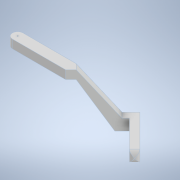
# Autodesk Inventor part: connector
Saved by Autodesk Inventor 2022 (Build 260153000, 153)
## iProperties
Created: 2023-07-22
Part Number: connector
Material: Generic
Document SubType Name: Modeling
Designer: Eric Cao
Density: 1 g/cm^3
Appearance: Plate - Blue
Author: Eric Cao
Autodesk Inventor part; units mm, degrees
ref_plane "YZ Plane" through (0, 0, 0) normal (1, 0, 0) x (0, 1, 0)
ref_plane "XZ Plane" through (0, 0, 0) normal (0, 1, 0) x (-1, 0, 0)
ref_plane "XY Plane" through (0, 0, 0) normal (0, 0, 1) x (1, 0, 0)
sketch "Sketch1" plane through (0, 0, 0) normal (0, 1, 0) x (-1, 0, 0)
  line L0 (0, 0) -> (50, 0)
  arc A0 (50, -10) -> (50, 0) centre (50, -5) ccw
  line L1 (50, -10) -> (0, -10)
  line L2 (0, -10) -> (-30, -40)
  line L3 (-30, -40) -> (-60, -10)
  arc A1 (-55.0192, -4.9808) -> (-60, -10) centre (-57.5, -7.5) ccw
  line L4 (-55.0192, -4.9808) -> (-30, -30)
  line L5 (-30, -30) -> (0, 0)
  dimension "d0" = 10
  dimension "d1" = 5
  dimension "d2" = 50
  dimension "d4" = 135
  dimension "d5" = 50
  dimension "d6" = 135
  dimension "d7" = 30
  dimension "d9" = 90
  dimension "d10" = 3.5356
  dimension "d40" = 30
  constraints: 12 end point, 4 point on circle, 2 centre point
  measures "d0" distance between parallel lines of L1 L0
  measures "d1" radius of A0
  measures "d2" horizontal distance of L0.start A0.centre
  measures "d4" angle of L2 L1
  measures "d5" distance of L1.end L1.start
  measures "d6" angle of L0 L5
  measures "d7" horizontal distance of L1.end L2.end
  measures "d9" angle of L4 L5
  measures "d10" radius of A1
  measures "d40" horizontal distance of L0.start L4.end
extrude "Extrusion1" add sketch "Sketch1" against normal blind 50
sketch "Sketch2" plane through (-50, 0, 0) normal (0, 0, 1) x (1, 0, 0)
  line L0 (-5, 0) -> (-5, -50) projected
  line L1 (80, -50) -> (50, -50) projected
  line L2 (-5, -8) -> (50, -8)
  line L3 (50, -8) -> (50, -50)
  line L4 (50, -50) -> (-5, -50)
  line L5 (-5, -50) -> (-5, -8)
  line L6 (0, 0) -> (50, 0) projected
  dimension "d13" = 8
  constraints: 8 end point, 2 parallel, 1 horizontal, 1 perpendicular, 1 point on line
  measures "d13" distance between parallel lines of L6 L2
extrude "Extrusion2" cut sketch "Sketch2" against normal blind 50
sketch "Sketch3" plane through (-50, -8, 0) normal (0, -1, 0) x (1, 0, 0)
  line L0 (0, 0) -> (50, 0) projected
  arc A0 (0, 0) -> (0, -10) centre (0, -5) ccw projected
  circle A1 centre (0, -5) radius 3
  dimension "d19" = 3
  constraints: 1 centre point, 1 coincident
  measures "d19" radius of A1
extrude "Extrusion3" cut sketch "Sketch3" against normal blind 5
sketch "Sketch4" plane through (-50, -3, -5) normal (0, -1, 0) x (1, 0, 0)
  circle A0 centre (0, 0) radius 0.525
  point P0 (50, 5)
  dimension "d22" = 1.05
  constraints: 1 centre point
  measures "d22" diameter of A0
extrude "Extrusion4" cut sketch "Sketch4" against normal blind 5
sketch "Sketch5" plane through (30, -50, -40) normal (-0.7071068, 0, -0.7071068) x (-0.7071068, 0, 0.7071068)
  line L0 (42.4264, 42) -> (77.7817, 42) projected
  line L1 (42.4264, 42) -> (16.7059, 0)
  line L2 (42.4264, 0) -> (0, 0) projected
  line L3 (16.7059, 0) -> (42.4264, 0)
  line L4 (42.4264, 0) -> (42.4264, 42)
  line L5 (42.4264, 42) -> (42.4264, 0) projected
  line L6 (7.0711, 50) -> (7.0711, 0) projected
  line L7 (0, 50) -> (42.4264, 50) projected
  line L8 (7.0711, 50) -> (42.4264, 50)
  line L9 (42.4264, 50) -> (11.8774, 10.4177)
  line L10 (11.8774, 10.4177) -> (7.0711, 10.4177)
  line L11 (7.0711, 10.4177) -> (7.0711, 50)
  point P0 (49.4975, 50)
  point P1 (7.0711, 10.4177)
  dimension "d41" = 50
  constraints: 14 end point, 3 point on line, 1 collinear, 1 horizontal, 1 parallel, 1 perpendicular
  measures "d41" distance of L7.end L9.end
extrude "Extrusion5" cut sketch "Sketch5" against normal through all
sketch "Sketch7" plane through (0, -50, 0) normal (0.7071068, 0, 0.7071068) x (0.7071068, 0, -0.7071068)
  line L0 (0, 42) -> (7.0711, 42) projected
  line L1 (7.0711, 0) -> (7.0711, 42) projected
  line L2 (0, 42) -> (7.0711, 42)
  line L3 (7.0711, 42) -> (7.0711, 0)
  line L4 (7.0711, 0) -> (0, 0)
  line L5 (0, 0) -> (0, 42)
  point P0 (0, 50)
  constraints: 8 end point, 2 parallel, 1 horizontal, 1 perpendicular
extrude "Extrusion6" cut sketch "Sketch7" against normal through all
sketch "Sketch8" plane through (55.0192, -50, -4.9808) normal (-0.7071068, 0, 0.7071068) x (0.7071068, 0, 0.7071068)
  line L0 (-42.4536, 10.4177) -> (-42.4536, 50) projected
  line L1 (-42.4536, 10.4177) -> (3.5084, 10.4177)
  line L2 (3.5084, 10.4177) -> (3.5084, 50.93)
  line L3 (3.5084, 50.93) -> (-42.4536, 50.93)
  line L4 (-42.4536, 50.93) -> (-42.4536, 10.4177)
  point P0 (-35.3825, 50)
  point P1 (-42.4536, 50)
  point P2 (-42.4536, 14.8933)
  point P3 (-42.4536, 14.8933)
  constraints: 8 end point, 2 parallel, 1 horizontal, 1 perpendicular
extrude "Extrusion7" cut sketch "Sketch8" against normal blind 10
sketch "Sketch9" plane through (30, -50, -30) normal (-0.7071068, 0, 0.7071068) x (0.7071068, 0, 0.7071068)
  line L0 (-7.0711, 0) -> (35.3553, 0) projected
  line L1 (35.3553, 10.4177) -> (35.3553, 0) projected
  arc A0 (35.3553, 0) -> (35.3553, 10.4177) centre (33.2861, 5.2088) ccw
  line L2 (38.8909, 10.4177) -> (38.8909, 0) projected
  line L3 (35.3825, 10.4177) -> (35.3825, 0) projected
  line L4 (35.3825, 10.4177) -> (38.8909, 10.4177)
  line L5 (35.3553, 0) -> (38.8909, 0) projected
  line L6 (38.8909, 0) -> (38.8909, 10.4177)
  line L7 (38.8909, 0) -> (35.3553, 0)
  point P0 (0, 50)
  point P1 (35.3825, 10.4068)
  point P2 (38.8909, 5.2088)
  point P3 (35.3825, 0.0109)
  constraints: 6 end point, 2 horizontal, 2 point on circle, 1 centre point, 1 collinear, 1 tangent
extrude "Extrusion8" cut sketch "Sketch9" against normal blind 10 contours L3 L4 L2 A0 | A0 L2 L5 L3
sketch "Sketch10" plane through (30, -50, -30) normal (-0.7071068, 0, 0.7071068) x (0.7071068, 0, 0.7071068)
  line L0 (35.3825, 10.4177) -> (0, 10.4177) projected
  circle A0 centre (33.2768, 5.2087) radius 2.5
  point P0 (0, 50)
  dimension "d33" = 5.209
  dimension "d34" = 2.5
  constraints: 1 centre point, 1 coincident
  measures "d33" distance from line of L0 point (33.277, 5.209)
  measures "d34" radius of A0
extrude "Extrusion9" cut sketch "Sketch10" against normal blind 5
sketch "Sketch11" plane through (57.0658, -44.7913, -10.0053) normal (-0.7071068, 0, 0.7071068) x (0.7071068, 0, 0.7071068)
  circle A0 centre (0, 0) radius 1.05
  point P0 (-33.2768, 44.7913)
  dimension "d37" = 1.05
  constraints: 1 centre point
  measures "d37" radius of A0
extrude "Extrusion10" cut sketch "Sketch11" against normal blind 11
body "Solid1"
